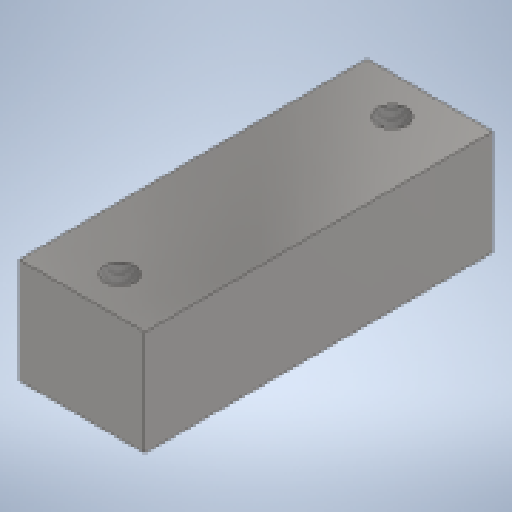
# Autodesk Inventor part: Pillow_support
Saved by Autodesk Inventor 2025.2 (Build 292293000, 293)
## iProperties
Created: 2025-02-20
Part Number: Pillow_support
Material: Stainless Steel
Document SubType Name: Modeling
Designer: Sergio Quintero
Density: 8 g/cm^3
Appearance: Semi-Polished
Mass: 462.731 g
Surface Area: 113.199 cm^2
Volume: 57.8414 cm^3
Author: Sergio Quintero
Autodesk Inventor part; units mm, degrees
ref_plane "YZ Plane" through (0, 0, 0) normal (1, 0, 0) x (0, 1, 0)
ref_plane "XZ Plane" through (0, 0, 0) normal (0, 1, 0) x (-1, 0, 0)
ref_plane "XY Plane" through (0, 0, 0) normal (0, 0, 1) x (1, 0, 0)
sketch "Sketch1" plane through (0, 0, 0) normal (0, 1, 0) x (-1, 0, 0)
  line L0 (-15, -41.5) -> (15, -41.5)
  line L1 (15, -41.5) -> (15, 41.5)
  line L2 (15, 41.5) -> (-15, 41.5)
  line L3 (-15, 41.5) -> (-15, -41.5)
  line L4 (-15, -41.5) -> (15, 41.5) construction
  line L5 (15, -41.5) -> (-15, 41.5) construction
  point P0 (0, 0)
  dimension "d0" = 30
  dimension "d1" = 83
  constraints: 12 end point, 2 midpoint, 2 parallel, 1 horizontal, 1 perpendicular
  measures "d0" distance of L2.end L1.end
  measures "d1" distance of L1.end L0.end
extrude "Extrusion1" add sketch "Sketch1" along normal blind 25
sketch "Sketch2" plane through (0, 25, 0) normal (0, 1, 0) x (1, 0, 0)
  line L0 (-15, 41.5) -> (-15, -41.5) projected
  line L1 (-15, -41.5) -> (15, -41.5) projected
  point P0 (0, 0)
  point P1 (0, -32.5)
  point P2 (0, 32.5)
  dimension "d4" = 15
  dimension "d6" = 9
  dimension "d14" = 65
  dimension "d15" = 15
  measures "d4" distance from line of point (0, -32.5) L0
  measures "d6" distance from line of L1 point (0, -32.5)
  measures "d14" distance of point (0, 32.5) point (0, -32.5)
  measures "d15" distance from line of L0 point (0, 32.5)
hole "Hole1" at (0, 25, 32.5) at (0, 25, -32.5) direction (0, -1, 0) diameter 7.134 end through all thread size "M8x0.8" class "6H" standard "ISO Metric profile"
body "Solid1"
